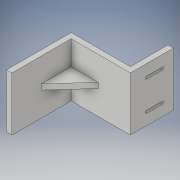
# Autodesk Inventor part: Bracket for door
Saved by Autodesk Inventor 2017 (Build 210142000, 142)
## iProperties
Created: 2018-12-15
Part Number: Bracket for door
Material: Generic
Document SubType Name: Modeling
Designer: Mitch
Density: 1 g/cm^3
Appearance: Default
Author: Mitch
Autodesk Inventor part; units mm, degrees
ref_plane "YZ Plane" through (0, 0, 0) normal (1, 0, 0) x (0, 1, 0)
ref_plane "XY Plane" through (0, 0, 0) normal (0, 0, 1) x (1, 0, 0)
sketch "Sketch1" plane through (0, 0, 0) normal (0, 1, 0) x (-1, 0, 0)
  line L0 (0, 0) -> (69.85, 0)
  line L1 (69.85, 0) -> (69.85, 69.85)
  line L2 (69.85, 69.85) -> (76.2, 69.85)
  line L3 (76.2, 69.85) -> (76.2, -6.35)
  line L4 (76.2, -6.35) -> (6.35, -6.35)
  line L5 (6.35, -6.35) -> (6.35, -50.8)
  line L6 (6.35, -50.8) -> (0, -50.8)
  line L7 (0, -50.8) -> (0, 0)
  dimension "d0" = 69.85
  dimension "d1" = 6.35
  dimension "d2" = 6.35
  dimension "d3" = 76.2
  dimension "d4" = 50.8
  dimension "d5" = 6.35
  constraints: 16 end point, 7 perpendicular, 1 horizontal
  measures "d0" distance of L0.start L0.end
  measures "d1" distance of L1.end L2.end
  measures "d2" distance between parallel lines of L0 L4
  measures "d3" distance of L2.end L3.end
  measures "d4" distance of L6.end L0.start
  measures "d5" distance between parallel lines of L7 L5
extrude "Extrusion1" add sketch "Sketch1" along normal blind 63.5
ref_plane "Work Plane1" through (0, 31.75, 0) normal (0, 1, 0) x (-1, 0, 0)
sketch "Sketch2" plane through (0, 31.75, 0) normal (0, 1, 0) x (-1, 0, 0)
  line L0 (36.2295, -8.0729) -> (10.8295, -35.6388)
  point P0 (0, 0)
  dimension "d27" = 25.4
  constraints: 2 end point
  measures "d27" horizontal distance of L0.start L0.end
extrude "Rib1" add sketch "Sketch2" along normal mid plane 6.35 rib yes fills toward (23.4927, -21.8219) open curves L0
sketch "Sketch3" plane through (0, 31.75, 0) normal (0, 1, 0) x (-1, 0, 0)
  line L0 (40.2992, 2.5373) -> (62.2373, 26.7221)
  point P0 (0, 0)
  constraints: 2 end point
extrude "Rib2" add sketch "Sketch3" along normal mid plane 6.35 rib yes fills toward (51.3053, 14.5961) open curves L0
sketch "Sketch4" plane through (-6.35, 0, -50.8) normal (-1, 0, 0) x (0, 0, 1)
  line L0 (31.75, 12.827) -> (12.7, 12.827)
  line L1 (12.7, 12.827) -> (12.7, 15.748)
  line L2 (12.7, 15.748) -> (31.75, 15.748)
  line L3 (31.75, 15.748) -> (31.75, 12.827)
  line L4 (44.45, 0) -> (0, 0) projected
  line L5 (0, 0) -> (0, 63.5) projected
  arc A0 (31.75, 12.827) -> (31.75, 15.748) centre (31.75, 14.2875) ccw
  arc A1 (12.7, 15.748) -> (12.7, 12.827) centre (12.7, 14.2875) ccw
  line L6 (0, 31.75) -> (68.349, 31.75)
  line L7 (31.75, 50.673) -> (12.7, 50.673)
  line L8 (12.7, 50.673) -> (12.7, 47.752)
  line L9 (12.7, 47.752) -> (31.75, 47.752)
  line L10 (31.75, 47.752) -> (31.75, 50.673)
  arc A2 (31.75, 47.752) -> (31.75, 50.673) centre (31.75, 49.2125) ccw
  arc A3 (12.7, 50.673) -> (12.7, 47.752) centre (12.7, 49.2125) ccw
  point P0 (50.8, 0)
  dimension "d21" = 12.827
  dimension "d22" = 12.7
  dimension "d23" = 2.921
  dimension "d24" = 19.05
  constraints: 18 end point, 8 point on circle, 6 symmetric about line, 4 centre point, 3 midpoint, 2 horizontal, 2 parallel, 1 perpendicular, 2 other
  measures "d21" distance between parallel lines of L4 L0
  measures "d22" distance between parallel lines of L5 L1
  measures "d23" distance of L2.end L0.start
  measures "d24" distance of L1.end L2.end
extrude "Extrusion2" cut sketch "Sketch4" against normal blind 63.5
body "Solid1"
